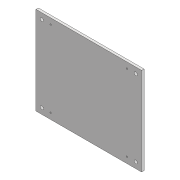
# Autodesk Inventor part: MTLV-M02
Saved by Autodesk Inventor 2020 (Build 240168000, 168)
## iProperties
Created: 2020-03-27
Part Number: MTLV-M02
Material: Generic
Document SubType Name: Modeling
Designer: John K
Density: 1 g/cm^3
Appearance: Default
Author: John K
Autodesk Inventor part; units mm, degrees
ref_plane "YZ Plane" through (0, 0, 0) normal (1, 0, 0) x (0, 1, 0)
ref_plane "XZ Plane" through (0, 0, 0) normal (0, 1, 0) x (-1, 0, 0)
ref_plane "XY Plane" through (0, 0, 0) normal (0, 0, 1) x (1, 0, 0)
sketch "Sketch1" plane through (0, 0, 0) normal (0, 0, 1) x (1, 0, 0)
  line L0 (-90, -75) -> (90, -75)
  line L1 (90, -75) -> (90, 75)
  line L2 (90, 75) -> (-90, 75)
  line L3 (-90, 75) -> (-90, -75)
  line L4 (-90, -75) -> (90, 75) construction
  line L5 (90, -75) -> (-90, 75) construction
  point P0 (0, 0)
  dimension "d0" = 180
  dimension "d1" = 150
  constraints: 12 end point, 2 midpoint, 2 parallel, 1 horizontal, 1 perpendicular
  measures "d0" distance of L1.end L2.end
  measures "d1" distance of L0.end L1.end
extrude "Extrusion1" add sketch "Sketch1" along normal blind 4.1
sketch "Sketch2" plane through (0, 0, 4.1) normal (0, 0, 1) x (1, 0, 0)
  line L0 (90, 75) -> (-90, 75) projected
  line L1 (-90, 75) -> (-90, -75) projected
  line L2 (-90, -75) -> (90, -75) projected
  line L3 (90, -75) -> (90, 75) projected
  point P0 (0, 0)
  point P1 (-80, 65)
  point P2 (80, 65)
  point P3 (80, -65)
  point P4 (-80, -65)
  dimension "d4" = 10
  dimension "d5" = 10
  dimension "d6" = 10
  dimension "d7" = 10
  constraints: 2 horizontal alignment, 2 vertical alignment
  measures "d4" distance from line of point (-80, 65) L0
  measures "d5" distance from line of point (-80, 65) L1
  measures "d6" distance from line of point (-80, -65) L2
  measures "d7" distance from line of point (80, 65) L3
hole "Hole1" at (-80, 65, 4.1) at (80, 65, 4.1) at (80, -65, 4.1) at (-80, -65, 4.1) direction (0, 0, -1) diameter 5.5 depth 9.1 tip angle 118 clearance for "Flat Head Machine Screw" size "M5" standard "Ansi Metric M Profile"
sketch "Sketch3" plane through (0, 0, 4.1) normal (0, 0, 1) x (1, 0, 0)
  circle A0 centre (-80, 65) radius 2.75 projected
  circle A1 centre (80, 65) radius 2.75 projected
  circle A2 centre (-80, -65) radius 2.75 projected
  point P0 (0, 0)
  point P1 (-65, 65)
  point P2 (65, 65)
  point P3 (65, -65)
  point P4 (-65, -65)
  dimension "d15" = 15
  dimension "d16" = 15
  constraints: 4 horizontal alignment, 2 vertical alignment
  measures "d15" distance of point (-65, 65) A0.centre
  measures "d16" distance of A1.centre point (65, 65)
hole "Hole2" at (-65, 65, 4.1) at (65, 65, 4.1) at (65, -65, 4.1) at (-65, -65, 4.1) direction (0, 0, -1) diameter 2.459 depth 8.8 tip angle 118 thread size "M3x0.5" class "6H" standard "ANSI Metric M Profile"
equation "\"d5\" = d4"
equation "\"d6\" = d4"
equation "\"d7\" = d4"
equation "\"d16\" = d15"
body "Solid1"
